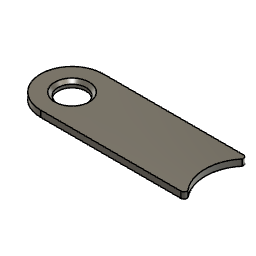
Poussoir v1 (Autodesk Fusion 360 design; units mm, degrees)
Autodesk Fusion 360 part; units mm, degrees
sketch "Sketch1" plane through (0, 0, 0) normal (0, 1, 0) x (1, 0, 0)
  line L0 (17.4087, -54.8067) -> (135.0065, -54.8067) construction
  circle A0 centre (37.1699, -54.8067) radius 10
  line L1 (9.2396, -44.8067) -> (81.8771, -44.8067) construction
  line L2 (13.4192, -64.8067) -> (138.6161, -64.8067) construction
  circle A1 centre (37.1699, -54.8067) radius 4.5
  circle A2 centre (37.1699, -54.8067) radius 7.5 construction
  line L3 (44.6699, -37.6811) -> (44.6699, -71.7825) construction
  line L4 (46.6699, -36.8465) -> (46.6699, -73.6307) construction
  line L5 (79.6699, -35.9522) -> (79.6699, -73.0345) construction
  line L6 (93.1699, -35.833) -> (93.1699, -73.7499) construction
  circle A3 centre (93.1699, -54.7914) radius 13.5
  line L7 (37.1699, -44.8067) -> (84.084, -44.8067)
  line L8 (37.1699, -64.8067) -> (81.9057, -64.8067)
  line L9 (82.084, -39.2431) -> (82.084, -68.9507) construction
  line L10 (82.6289, -46.466) -> (82.084, -47.0874)
  line L11 (82.6565, -63.1461) -> (82.084, -62.4955)
  arc A4 (82.6289, -46.466) -> (81.8771, -44.8067) centre (81.8771, -45.8067) ccw
  arc A5 (81.9057, -64.8067) -> (82.6565, -63.1461) centre (81.9057, -63.8067) ccw
  dimension "d1" = 20
  dimension "d2" = 9
  dimension "d3" = 15
  dimension "d4" = 2
  dimension "d5" = 33
  dimension "d6" = 13.5
  dimension "d7" = 27
  dimension "d8" = 2
  dimension "d9" = 1
  dimension "d10" = 1
  constraint horizontal L0
  constraint coincident L0 A0.centre
  constraint horizontal L1
  constraint horizontal L2
  constraint tangent A0 L1
  constraint tangent A0 L2
  constraint concentric A0 A1
  constraint concentric A1 A2
  constraint perpendicular L2 L3
  constraint tangent A2 L3
  constraint perpendicular L2 L4
  constraint perpendicular L0 L5
  constraint vertical L6
  constraint midpoint L6 A3.centre
  constraint coincident A0 L7.start
  constraint coincident L1 L7.start
  constraint coincident L1 L7.end
  constraint coincident A3 L7.end
  constraint coincident A0 L8.start
  constraint tangent A0 L8
  constraint perpendicular L2 L9
  constraint coincident A3 L10.end
  constraint coincident L9 L10.end
  constraint coincident A3 L11.end
  constraint coincident L9 L11.end
  constraint coincident L7.end L10
  constraint tangent L1 A4
  constraint tangent L10 A4
  constraint tangent L8 A5
  constraint tangent L11 A5
  measures "d1" diameter of A0
  measures "d2" diameter of A1
  measures "d3" diameter of A2
  measures "d4" distance of L3 L4
  measures "d5" distance of L4 L5
  measures "d6" distance of L5 L6
  measures "d7" diameter of A3
  measures "d8" distance of L7.end L9
  measures "d9" radius of A4
  measures "d10" radius of A5
extrude "Extrude1" add sketch "Sketch1" along normal blind 2 contours A0 | A0 A3 L7 L8 A4 A5
chamfer "Chamfer1" distance 1 angle 45 1 edges at (32.9745, 2, 53.1794)
equation "d6 = ( 27 / 2 ) * 1 mm"
